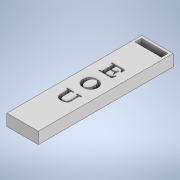
# Autodesk Inventor part: LegWithTextEOU
Saved by Autodesk Inventor 2021 (Build 250183000, 183)
## iProperties
Created: 2024-05-05
Part Number: LegWithTextEOU
Material: Generic
Document SubType Name: Modeling
Designer: brybr
Density: 1 g/cm^3
Appearance: Default
Author: brybr
Autodesk Inventor part; units mm, degrees
ref_plane "YZ Plane" through (0, 0, 0) normal (1, 0, 0) x (0, 1, 0)
ref_plane "XZ Plane" through (0, 0, 0) normal (0, 1, 0) x (-1, 0, 0)
ref_plane "XY Plane" through (0, 0, 0) normal (0, 0, 1) x (1, 0, 0)
sketch "Sketch1" plane through (0, 0, 0) normal (0, 0, 1) x (1, 0, 0)
  line L0 (-17.5, 6.5) -> (17.5, 6.5)
  line L1 (17.5, 6.5) -> (17.5, -6.5)
  line L2 (17.5, -6.5) -> (-17.5, -6.5)
  line L3 (-17.5, -6.5) -> (-17.5, 6.5)
  line L4 (-17.5, 6.5) -> (17.5, -6.5) construction
  line L5 (17.5, 6.5) -> (-17.5, -6.5) construction
  line L6 (-17.5, 6.5) -> (17.5, 6.5) construction
  point P0 (0, 0)
  dimension "d0" = 35
  dimension "d1" = 0
  dimension "d2" = 13
  constraints: 14 end point, 2 horizontal, 2 midpoint, 2 parallel, 1 collinear, 1 perpendicular
  measures "d0" distance of L0.start L0.end
  measures "d1" distance between parallel lines of L0 L6
  measures "d2" distance of L0.end L1.end
extrude "Extrusion1" add sketch "Sketch1" along normal blind 150
sketch "Sketch2" plane through (-17.5, 6.5, 0) normal (0, 1, 0) x (1, 0, 0)
  line L0 (2.8, -10.2) -> (32.2, -10.2)
  line L1 (32.2, -10.2) -> (32.2, -3)
  line L2 (32.2, -3) -> (2.8, -3)
  line L3 (2.8, -3) -> (2.8, -10.2)
  line L4 (2.8, -10.2) -> (32.2, -3) construction
  line L5 (32.2, -10.2) -> (2.8, -3) construction
  line L6 (2.8, -10.2) -> (32.2, -10.2) construction
  line L7 (2.8, -6.6) -> (0, -6.6)
  line L8 (0, 0) -> (0, -150) projected
  line L9 (35, 0) -> (35, -150) projected
  line L10 (35, -6.6) -> (32.2, -6.6)
  line L11 (35, 0) -> (0, 0) projected
  line L12 (35, -150) -> (0, -150) projected
  point P0 (17.5, 0)
  point P1 (17.5, -6.6)
  dimension "d6" = 29.4
  dimension "d7" = 0
  dimension "d8" = 7.2
  dimension "d9" = 3
  constraints: 18 end point, 4 midpoint, 3 horizontal, 3 point on line, 2 collinear, 2 parallel, 1 perpendicular
  measures "d6" distance of L0.start L0.end
  measures "d7" distance between parallel lines of L0 L6
  measures "d8" distance of L1.end L0.end
  measures "d9" distance between parallel lines of L11 L2
extrude "Extrusion2" cut sketch "Sketch2" against normal through all contours L3 L2 L1 L0
sketch "Sketch3" plane through (-17.5, 6.5, 0) normal (0, 1, 0) x (1, 0, 0)
  line L0 (6.4393, -10.6292) -> (29.4313, -10.6292) construction
  line L1 (29.4313, -10.6292) -> (29.4313, -139.9049) construction
  line L2 (29.4313, -139.9049) -> (6.4393, -139.9049) construction
  line L3 (6.4393, -139.9049) -> (6.4393, -10.6292) construction
  spline S0 degree 2 poles (10.0603, -42.9745) (10.7198, -43.0132) (11.1982, -43.0779) knots 0 0 0 1 1 1
  spline S1 degree 2 poles (11.1982, -43.0779) (12.1034, -43.2072) (13.306, -43.2072) knots 0 0 0 1 1 1
  spline S2 degree 2 poles (13.306, -43.2072) (13.7198, -43.2072) (15.4267, -43.1426) knots 0 0 0 1 1 1
  spline S3 degree 2 poles (15.4267, -43.1426) (17.987, -43.0391) (20.056, -43.0391) knots 0 0 0 1 1 1
  line L4 (20.056, -43.0391) -> (22.1379, -43.0132)
  spline S4 degree 2 poles (22.1379, -43.0132) (22.8361, -43.0132) (24.2068, -43.1813) knots 0 0 0 1 1 1
  spline S5 degree 2 poles (24.2068, -43.1813) (24.4137, -43.4141) (24.4137, -43.802) knots 0 0 0 1 1 1
  line L5 (24.4137, -43.802) -> (24.4137, -46.1813)
  line L6 (24.4137, -46.1813) -> (24.4396, -46.6469)
  spline S6 degree 2 poles (24.4396, -46.6469) (24.4396, -46.7245) (24.4267, -46.8538) knots 0 0 0 1 1 1
  line L7 (24.4267, -46.8538) -> (23.9482, -46.8796)
  spline S7 degree 2 poles (23.9482, -46.8796) (23.8577, -46.8796) (23.5603, -46.8538) knots 0 0 0 1 1 1
  spline S8 degree 2 poles (23.5603, -46.8538) (23.4568, -46.621) (23.2887, -46.1813) knots 0 0 0 1 1 1
  line L8 (23.2887, -46.1813) -> (22.8361, -45.3667)
  spline S9 degree 2 poles (22.8361, -45.3667) (22.5646, -44.8495) (22.0991, -44.3063) knots 0 0 0 1 1 1
  spline S10 degree 2 poles (22.0991, -44.3063) (21.8146, -44.2288) (21.362, -44.2158) knots 0 0 0 1 1 1
  spline S11 degree 2 poles (21.362, -44.2158) (21.2456, -44.2029) (20.6637, -44.1512) knots 0 0 0 1 1 1
  spline S12 degree 2 poles (20.6637, -44.1512) (19.5905, -44.0607) (18.362, -44.0607) knots 0 0 0 1 1 1
  spline S13 degree 2 poles (18.362, -44.0607) (16.9655, -44.0607) (15.8534, -44.1124) knots 0 0 0 1 1 1
  spline S14 degree 2 poles (15.8534, -44.1124) (15.8275, -44.3969) (15.8275, -46.3753) knots 0 0 0 1 1 1
  line L9 (15.8275, -46.3753) -> (15.8275, -48.302)
  line L10 (15.8275, -48.302) -> (15.8275, -49.7374)
  spline S15 degree 2 poles (15.8275, -49.7374) (16.1249, -49.7762) (16.3318, -49.7762) knots 0 0 0 1 1 1
  spline S16 degree 2 poles (16.3318, -49.7762) (18.4008, -49.7762) (20.1465, -49.621) (20.5603, -49.3236) (20.7284, -48.9745) knots 0 0 0 1 2 3 3 3
  spline S17 degree 2 poles (20.7284, -48.9745) (20.8318, -48.7158) (21.1292, -47.2805) knots 0 0 0 1 1 1
  line L11 (21.1292, -47.2805) -> (21.2844, -47.2676)
  line L12 (21.2844, -47.2676) -> (21.9439, -47.2805)
  spline S18 degree 2 poles (21.9439, -47.2805) (21.9956, -48.302) (21.9956, -48.8322) knots 0 0 0 1 1 1
  spline S19 degree 2 poles (21.9956, -48.8322) (21.9956, -50.0348) (21.9568, -50.7331) (21.9568, -50.927) knots 0 0 0 1 2 2 2
  spline S20 degree 2 poles (21.9568, -50.927) (21.9568, -51.2374) (22.0215, -52.6081) (22.0215, -52.9313) knots 0 0 0 1 2 2 2
  line L13 (22.0215, -52.9313) -> (22.0215, -53.19)
  line L14 (22.0215, -53.19) -> (21.2068, -53.19)
  spline S21 degree 2 poles (21.2068, -53.19) (21.1551, -53.0089) (21.0387, -52.427) knots 0 0 0 1 1 1
  spline S22 degree 2 poles (21.0387, -52.427) (20.806, -51.3667) (20.6249, -51.0951) knots 0 0 0 1 1 1
  spline S23 degree 2 poles (20.6249, -51.0951) (20.4827, -50.8882) (20.1594, -50.7848) knots 0 0 0 1 1 1
  spline S24 degree 2 poles (20.1594, -50.7848) (19.9267, -50.7072) (18.4525, -50.7072) knots 0 0 0 1 1 1
  spline S25 degree 2 poles (18.4525, -50.7072) (16.7068, -50.7072) (15.8275, -50.7977) knots 0 0 0 1 1 1
  spline S26 degree 2 poles (15.8275, -50.7977) (15.8275, -51.0951) (15.8275, -51.1857) knots 0 0 0 1 1 1
  spline S27 degree 2 poles (15.8275, -51.1857) (15.8275, -52.5563) (15.8792, -53.4615) knots 0 0 0 1 1 1
  line L15 (15.8792, -53.4615) -> (15.8534, -55.9443)
  spline S28 degree 2 poles (15.8534, -55.9443) (15.8534, -56.3839) (16.1637, -56.5391) knots 0 0 0 1 1 1
  spline S29 degree 2 poles (16.1637, -56.5391) (16.6422, -56.7848) (19.0473, -56.7848) knots 0 0 0 1 1 1
  spline S30 degree 2 poles (19.0473, -56.7848) (20.6508, -56.7848) (21.7629, -56.5391) knots 0 0 0 1 1 1
  spline S31 degree 2 poles (21.7629, -56.5391) (22.5258, -56.371) (23.1206, -55.7762) knots 0 0 0 1 1 1
  spline S32 degree 2 poles (23.1206, -55.7762) (23.8965, -55.0003) (24.4137, -53.6167) knots 0 0 0 1 1 1
  spline S33 degree 2 poles (24.4137, -53.6167) (24.7758, -53.5779) (25.0086, -53.5779) knots 0 0 0 1 1 1
  spline S34 degree 2 poles (25.0086, -53.5779) (25.1249, -53.5779) (25.3836, -53.5908) knots 0 0 0 1 1 1
  spline S35 degree 2 poles (25.3836, -53.5908) (25.3448, -53.8753) (25.3318, -54.0693) knots 0 0 0 1 1 1
  line L16 (25.3318, -54.0693) -> (25.2542, -54.4184)
  line L17 (25.2542, -54.4184) -> (24.8405, -56.5908)
  line L18 (24.8405, -56.5908) -> (24.6336, -57.8969)
  spline S36 degree 2 poles (24.6336, -57.8969) (23.8836, -57.9357) (23.4439, -57.9357) knots 0 0 0 1 1 1
  spline S37 degree 2 poles (23.4439, -57.9357) (22.8103, -57.9357) (20.0172, -57.8193) knots 0 0 0 1 1 1
  spline S38 degree 2 poles (20.0172, -57.8193) (18.0517, -57.7417) (15.2715, -57.7417) knots 0 0 0 1 1 1
  spline S39 degree 2 poles (15.2715, -57.7417) (13.9008, -57.7417) (11.8836, -57.8581) knots 0 0 0 1 1 1
  line L19 (11.8836, -57.8581) -> (11.4051, -57.8581)
  line L20 (11.4051, -57.8581) -> (10.0086, -57.8969)
  line L21 (10.0086, -57.8969) -> (10.0086, -57.1081)
  spline S40 degree 2 poles (10.0086, -57.1081) (10.2284, -57.0563) (10.8879, -56.9788) knots 0 0 0 1 1 1
  spline S41 degree 2 poles (10.8879, -56.9788) (12.0775, -56.8495) (12.543, -56.6167) knots 0 0 0 1 1 1
  spline S42 degree 2 poles (12.543, -56.6167) (12.6594, -56.2805) (12.6594, -55.7762) knots 0 0 0 1 1 1
  spline S43 degree 2 poles (12.6594, -55.7762) (12.6594, -55.5822) (12.6465, -55.1038) knots 0 0 0 1 1 1
  line L22 (12.6465, -55.1038) -> (12.6594, -54.7546)
  line L23 (12.6594, -54.7546) -> (12.6206, -50.4227)
  line L24 (12.6206, -50.4227) -> (12.6336, -49.1296)
  line L25 (12.6336, -49.1296) -> (12.5818, -47.2805)
  line L26 (12.5818, -47.2805) -> (12.5948, -45.9874)
  line L27 (12.5948, -45.9874) -> (12.4913, -44.565)
  spline S44 degree 2 poles (12.4913, -44.565) (12.4913, -44.5132) (12.4655, -44.3322) knots 0 0 0 1 1 1
  spline S45 degree 2 poles (12.4655, -44.3322) (12.3491, -44.2029) (12.1292, -44.177) knots 0 0 0 1 1 1
  spline S46 degree 2 poles (12.1292, -44.177) (11.9999, -44.1512) (11.7801, -44.0995) knots 0 0 0 1 1 1
  spline S47 degree 2 poles (11.7801, -44.0995) (11.1206, -43.9701) (10.5129, -43.9443) knots 0 0 0 1 1 1
  spline S48 degree 2 poles (10.5129, -43.9443) (10.293, -43.9313) (10.0086, -43.8926) knots 0 0 0 1 1 1
  line L28 (10.0086, -43.8926) -> (10.0603, -42.9745)
  spline S49 degree 2 poles (9.653, -74.8921) (9.653, -73.4697) (10.209, -72.0343) knots 0 0 0 1 1 1
  spline S50 degree 2 poles (10.209, -72.0343) (10.6098, -70.9998) (12.0581, -69.2671) (14.2305, -67.9222) (16.5064, -67.3403) (17.903, -67.3403) knots 0 0 0 1 2 3 4 4 4
  spline S51 degree 2 poles (17.903, -67.3403) (20.2952, -67.3403) (23.8124, -69.1378) (24.8211, -70.6636) knots 0 0 0 1 2 2 2
  spline S52 degree 2 poles (24.8211, -70.6636) (26.1271, -72.655) (26.1271, -74.8274) knots 0 0 0 1 1 1
  spline S53 degree 2 poles (26.1271, -74.8274) (26.1271, -78.086) (21.7047, -82.7283) (17.7736, -82.7283) knots 0 0 0 1 2 2 2
  spline S54 degree 2 poles (17.7736, -82.7283) (16.7909, -82.7283) (15.9504, -82.599) knots 0 0 0 1 1 1
  spline S55 degree 2 poles (15.9504, -82.599) (15.3038, -82.5085) (14.8254, -82.3533) knots 0 0 0 1 1 1
  spline S56 degree 2 poles (14.8254, -82.3533) (13.9461, -82.0559) (13.8426, -82.0171) knots 0 0 0 1 1 1
  spline S57 degree 2 poles (13.8426, -82.0171) (12.5883, -81.3059) (11.0754, -79.8059) (10.5452, -78.8619) knots 0 0 0 1 2 2 2
  spline S58 degree 2 poles (10.5452, -78.8619) (10.2607, -78.3447) (9.8986, -76.961) knots 0 0 0 1 1 1
  spline S59 degree 2 poles (9.8986, -76.961) (9.653, -76.0688) (9.653, -74.8921) knots 0 0 0 1 1 1
  spline S60 degree 2 poles (17.4633, -68.4783) (16.4676, -68.4783) (14.9288, -69.4093) (14.5409, -69.9783) knots 0 0 0 1 2 2 2
  spline S61 degree 2 poles (14.5409, -69.9783) (13.8943, -70.9222) (13.3383, -73.1852) (13.3383, -74.8145) knots 0 0 0 1 2 2 2
  spline S62 degree 2 poles (13.3383, -74.8145) (13.3383, -75.7972) (13.4159, -76.224) knots 0 0 0 1 1 1
  spline S63 degree 2 poles (13.4159, -76.224) (13.4417, -76.3662) (13.4935, -76.6895) knots 0 0 0 1 1 1
  spline S64 degree 2 poles (13.4935, -76.6895) (13.5969, -77.5429) (13.7262, -77.9309) knots 0 0 0 1 1 1
  spline S65 degree 2 poles (13.7262, -77.9309) (14.2176, -79.3921) (14.4245, -79.7412) knots 0 0 0 1 1 1
  spline S66 degree 2 poles (14.4245, -79.7412) (14.7736, -80.3231) (15.4461, -80.905) knots 0 0 0 1 1 1
  spline S67 degree 2 poles (15.4461, -80.905) (15.7952, -81.2024) (17.1012, -81.6938) (17.7607, -81.6938) knots 0 0 0 1 2 2 2
  spline S68 degree 2 poles (17.7607, -81.6938) (18.9892, -81.6938) (21.1228, -80.53) (22.403, -77.7498) (22.403, -75.5257) knots 0 0 0 1 2 3 3 3
  spline S69 degree 2 poles (22.403, -75.5257) (22.403, -74.6076) (22.2736, -73.03) knots 0 0 0 1 1 1
  line L29 (22.2736, -73.03) -> (22.2219, -72.8102)
  spline S70 degree 2 poles (22.2219, -72.8102) (22.1831, -72.7197) (22.1055, -72.3447) knots 0 0 0 1 1 1
  spline S71 degree 2 poles (22.1055, -72.3447) (21.6788, -70.4567) (19.2866, -68.4783) (17.4633, -68.4783) knots 0 0 0 1 2 2 2
  line L30 (9.4267, -93.2709) -> (9.3879, -92.3657)
  spline S72 degree 2 poles (9.3879, -92.3657) (9.5948, -92.3528) (9.8146, -92.3528) knots 0 0 0 1 1 1
  spline S73 degree 2 poles (9.8146, -92.3528) (10.3965, -92.3528) (11.0301, -92.3916) knots 0 0 0 1 1 1
  spline S74 degree 2 poles (11.0301, -92.3916) (12.543, -92.4692) (12.8146, -92.4692) knots 0 0 0 1 1 1
  spline S75 degree 2 poles (12.8146, -92.4692) (13.7327, -92.4692) (15.4913, -92.3916) (16.862, -92.3787) (17.1077, -92.3657) knots 0 0 0 1 2 3 3 3
  line L31 (17.1077, -92.3657) -> (17.0948, -92.495)
  line L32 (17.0948, -92.495) -> (17.1206, -93.1675)
  line L33 (17.1206, -93.1675) -> (17.1206, -93.258)
  spline S76 degree 2 poles (17.1206, -93.258) (16.4741, -93.3614) (15.7887, -93.3614) knots 0 0 0 1 1 1
  spline S77 degree 2 poles (15.7887, -93.3614) (15.1422, -93.3614) (14.9353, -93.62) knots 0 0 0 1 1 1
  spline S78 degree 2 poles (14.9353, -93.62) (14.793, -93.7752) (14.793, -94.9778) knots 0 0 0 1 1 1
  spline S79 degree 2 poles (14.793, -94.9778) (14.793, -95.3528) (14.806, -95.5726) knots 0 0 0 1 1 1
  line L34 (14.806, -95.5726) -> (14.8189, -95.9864)
  line L35 (14.8189, -95.9864) -> (14.793, -97.0726)
  line L36 (14.793, -97.0726) -> (14.8706, -97.9907)
  line L37 (14.8706, -97.9907) -> (14.8189, -99.9692)
  line L38 (14.8189, -99.9692) -> (14.9741, -102.8528)
  spline S80 degree 2 poles (14.9741, -102.8528) (15.0258, -104.1071) (15.5172, -104.9347) knots 0 0 0 1 1 1
  spline S81 degree 2 poles (15.5172, -104.9347) (15.8922, -105.5425) (16.5517, -105.8916) knots 0 0 0 1 1 1
  spline S82 degree 2 poles (16.5517, -105.8916) (17.5215, -106.37) (18.4525, -106.37) knots 0 0 0 1 1 1
  spline S83 degree 2 poles (18.4525, -106.37) (19.5517, -106.37) (20.5086, -106.0856) knots 0 0 0 1 1 1
  spline S84 degree 2 poles (20.5086, -106.0856) (21.0646, -105.9175) (22.0732, -105.1933) (22.2672, -104.8959) knots 0 0 0 1 2 2 2
  spline S85 degree 2 poles (22.2672, -104.8959) (22.681, -104.2623) (22.8361, -103.7192) knots 0 0 0 1 1 1
  spline S86 degree 2 poles (22.8361, -103.7192) (23.056, -102.9562) (23.056, -101.3528) knots 0 0 0 1 1 1
  spline S87 degree 2 poles (23.056, -101.3528) (23.056, -98.5726) (22.7586, -95.0942) knots 0 0 0 1 1 1
  line L39 (22.7586, -95.0942) -> (22.7068, -94.4864)
  spline S88 degree 2 poles (22.7068, -94.4864) (22.668, -93.8011) (22.4611, -93.5812) knots 0 0 0 1 1 1
  spline S89 degree 2 poles (22.4611, -93.5812) (22.0861, -93.2192) (21.6336, -93.2192) knots 0 0 0 1 1 1
  line L40 (21.6336, -93.2192) -> (20.5603, -93.245)
  line L41 (20.5603, -93.245) -> (20.4051, -93.2062)
  line L42 (20.4051, -93.2062) -> (20.431, -92.3269)
  line L43 (20.431, -92.3269) -> (21.3361, -92.3269)
  line L44 (21.3361, -92.3269) -> (23.5344, -92.4304)
  spline S90 degree 2 poles (23.5344, -92.4304) (24.6336, -92.4304) (25.6422, -92.3269) knots 0 0 0 1 1 1
  line L45 (25.6422, -92.3269) -> (25.8361, -92.3528)
  spline S91 degree 2 poles (25.8361, -92.3528) (25.9008, -92.7278) (25.9008, -92.87) knots 0 0 0 1 1 1
  spline S92 degree 2 poles (25.9008, -92.87) (25.9008, -92.9993) (25.8491, -93.1804) knots 0 0 0 1 1 1
  spline S93 degree 2 poles (25.8491, -93.1804) (25.4353, -93.2968) (24.9568, -93.3226) knots 0 0 0 1 1 1
  spline S94 degree 2 poles (24.9568, -93.3226) (24.1939, -93.4261) (24.1034, -93.4907) knots 0 0 0 1 1 1
  spline S95 degree 2 poles (24.1034, -93.4907) (23.9482, -93.633) (23.9482, -93.9175) knots 0 0 0 1 1 1
  spline S96 degree 2 poles (23.9482, -93.9175) (23.9482, -94.1243) (23.987, -94.5123) knots 0 0 0 1 1 1
  spline S97 degree 2 poles (23.987, -94.5123) (24.0129, -94.8097) (24.0129, -95.5209) knots 0 0 0 1 1 1
  spline S98 degree 2 poles (24.0129, -95.5209) (24.0129, -95.9218) (24.0258, -96.3873) (24.0387, -96.62) knots 0 0 0 1 2 2 2
  spline S99 degree 2 poles (24.0387, -96.62) (24.0775, -97.4476) (24.0905, -98.3011) knots 0 0 0 1 1 1
  line L46 (24.0905, -98.3011) -> (24.2068, -100.6416)
  spline S100 degree 2 poles (24.2068, -100.6416) (24.2068, -102.9821) (23.8836, -104.5726) (23.612, -105.0252) knots 0 0 0 1 2 2 2
  spline S101 degree 2 poles (23.612, -105.0252) (23.1853, -105.7235) (21.6206, -106.8873) (19.2801, -107.5597) (17.7155, -107.5597) knots 0 0 0 1 2 3 3 3
  spline S102 degree 2 poles (17.7155, -107.5597) (15.931, -107.5597) (13.3706, -106.6028) (12.0775, -105.0511) (11.8318, -103.8226) knots 0 0 0 1 2 3 3 3
  spline S103 degree 2 poles (11.8318, -103.8226) (11.6637, -102.9692) (11.6637, -101.3787) knots 0 0 0 1 1 1
  line L47 (11.6637, -101.3787) -> (11.6637, -95.9088)
  spline S104 degree 2 poles (11.6637, -95.9088) (11.6637, -93.9692) (11.4827, -93.7106) knots 0 0 0 1 1 1
  spline S105 degree 2 poles (11.4827, -93.7106) (11.2241, -93.3614) (9.9051, -93.3097) knots 0 0 0 1 1 1
  spline S106 degree 2 poles (9.9051, -93.3097) (9.6206, -93.3097) (9.4267, -93.2709) knots 0 0 0 1 1 1
  point P0 (17.5, 0)
  constraints: 2 other
emboss "Emboss1" sketch "Sketch3" operation cut depth 20 direction (0, -1, 0)
sketch "Sketch4" plane through (3.3403, 6.5, 79.1677) normal (0, 1, 0) x (1, 0, 0)
  line L0 (-2.9374, 11.8274) -> (-2.096, 11.8274)
  line L1 (-2.096, 11.8274) -> (-2.096, -3.9827)
  line L2 (-2.096, -3.9827) -> (-2.9374, -3.9827)
  line L3 (-2.9374, -3.9827) -> (-2.9374, 11.8274)
  point P0 (-3.3403, 79.1677)
  constraints: 8 end point, 2 parallel, 1 horizontal, 1 perpendicular
extrude "Extrusion3" add sketch "Sketch4" against normal blind 13
body "Solid1"
